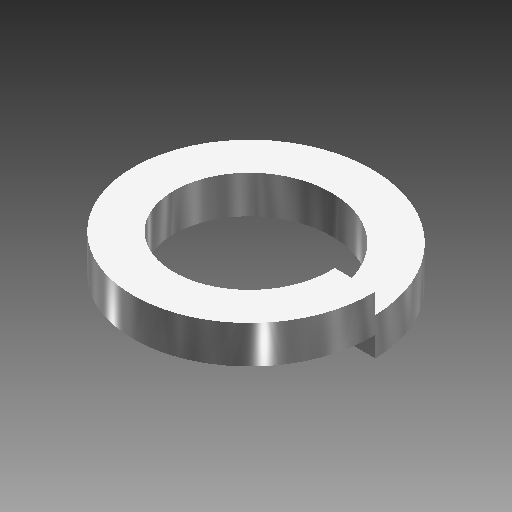
# Autodesk Inventor part: SSR-40 DA Lock Washer
Saved by Autodesk Inventor 2019 (Build 230136000, 136)
## iProperties
Created: 2014-11-01
Part Number: SSR-40 DA Lock Washer
Material: Nickel-Copper Alloy 400
Document SubType Name: Modeling
Designer: Tyler
Density: 8.83 g/cm^3
Appearance: Chrome - Polished
Mass: 0.131192 g
Surface Area: 0.61915 cm^2
Volume: 0.0148576 cm^3
Author: Tyler
Autodesk Inventor part; units mm, degrees
ref_plane "YZ Plane" through (0, 0, 0) normal (1, 0, 0) x (0, 1, 0)
ref_plane "XZ Plane" through (0, 0, 0) normal (0, 1, 0) x (-1, 0, 0)
ref_plane "XY Plane" through (0, 0, 0) normal (0, 0, 1) x (1, 0, 0)
sketch "Sketch1" plane through (0, 0, 0) normal (0, 0, 1) x (1, 0, 0)
  line L0 (0, 0) -> (0, 13.0773)
  line L1 (0, 0) -> (1.9685, 0)
  line L2 (2.9845, 0.4699) -> (1.9685, 0.4699)
  line L3 (1.9685, 0.4699) -> (1.9685, -0.4699)
  line L4 (1.9685, -0.4699) -> (2.9845, -0.4699)
  line L5 (2.9845, -0.4699) -> (2.9845, 0.4699)
  point P0 (2.9845, 0)
  dimension "d0" = 1.9685
  dimension "d1" = 0.9398
  dimension "d2" = 1.016
  constraints: 12 end point, 2 coincident, 2 horizontal, 2 midpoint, 2 parallel, 1 horizontal alignment, 1 perpendicular, 1 vertical
  measures "d0" distance of L0.start L1.end
  measures "d1" distance of L4.end L2.start
  measures "d2" distance of L2.start L2.end
coil "Coil1" sketch "Sketch1" operation add axis through (0, 0, 0) along (0, 1, 0) pitch 0.508 turns 1 hand right
body "Solid1"
